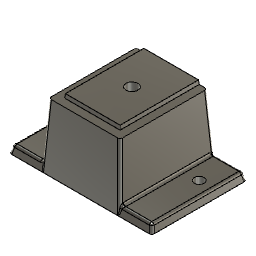
Mounting Base (Autodesk Fusion 360 design; units mm, degrees)
Autodesk Fusion 360 part; units mm, degrees
sketch "bottom" plane through (0, 0, 0) normal (0, 0, 1) x (1, 0, 0)
  line L0 (0, 0) -> (114.3, 0)
  line L1 (114.3, 0) -> (114.3, 76.2)
  line L2 (114.3, 76.2) -> (0, 76.2)
  line L3 (0, 76.2) -> (0, 0)
  line L4 (25.4, 76.2) -> (25.4, 0)
  line L5 (88.9, 0) -> (88.9, 76.2)
  line L6 (82.55, 6.35) -> (31.75, 6.35)
  line L7 (31.75, 69.85) -> (82.55, 69.85)
  line L8 (31.75, 69.85) -> (31.75, 6.35)
  line L9 (82.55, 6.35) -> (82.55, 69.85)
  circle A0 centre (12.7, 50.8) radius 3.9687
  circle A1 centre (101.6, 50.8) radius 3.9688
  dimension "d1" = 114.3
  dimension "d2" = 76.2
  dimension "d3" = 25.4
  dimension "d4" = 25.4
  dimension "d5" = 6.35
  dimension "d6" = 6.35
  dimension "d7" = 6.35
  dimension "d8" = 6.35
  dimension "d32" = 7.9375
  dimension "d33" = 7.9375
  dimension "d34" = 25.4
  dimension "d35" = 25.4
  dimension "d36" = 12.7
  dimension "d37" = 12.7
  constraint horizontal L0
  constraint vertical L1
  constraint horizontal L2
  constraint vertical L3
  constraint coincident L0.start L3.end
  constraint coincident L2 L4.start
  constraint coincident L0 L4.end
  constraint perpendicular L0 L4
  constraint coincident L0 L5.start
  constraint coincident L2 L5.end
  constraint perpendicular L2 L5
  constraint perpendicular L4 L6
  constraint perpendicular L5 L7
  constraint perpendicular L6 L8
  constraint perpendicular L7 L9
  measures "d1" distance of L0.start L0.end
  measures "d2" distance of L0.start L2.end
  measures "d3" distance of L3 L4
  measures "d4" distance of L1 L5
  measures "d5" distance of L2 L7
  measures "d6" distance of L0 L6
  measures "d7" distance of L4 L8
  measures "d8" distance of L5 L9
  measures "d32" diameter of A0
  measures "d33" diameter of A1
  measures "d34" distance of L2 A0.centre
  measures "d35" distance of L2 A1.centre
  measures "d36" distance of L3 A0.centre
  measures "d37" distance of L1 A1.centre
ref_plane "WorkPlane1" through (0, 0, 50.8) normal (0, 0, 1) x (1, 0, 0)
sketch "top" plane through (0, 0, 50.8) normal (0, 0, 1) x (1, 0, 0)
  line L0 (28.575, 73.025) -> (28.575, 3.175)
  line L1 (85.725, 3.175) -> (85.725, 73.025)
  line L2 (28.575, 73.025) -> (85.725, 73.025)
  line L3 (28.575, 3.175) -> (85.725, 3.175)
  line L4 (79.375, 73.025) -> (79.375, 9.525)
  line L5 (34.925, 73.025) -> (34.925, 9.525)
  line L6 (34.925, 9.525) -> (79.375, 9.525)
  circle A0 centre (57.15, 41.275) radius 4.7625
  dimension "d20" = 6.35
  dimension "d21" = 44.45
  dimension "d22" = 6.35
  dimension "d25" = 9.525
  dimension "d26" = 38.1
  dimension "d27" = 22.225
  constraint perpendicular L1 L2
  constraint perpendicular L1 L3
  constraint coincident L2 L4.start
  constraint perpendicular L3 L4
  constraint coincident L2 L5.start
  constraint perpendicular L3 L5
  constraint perpendicular L4 L6
  measures "d20" distance of L1 L4
  measures "d21" distance of L4 L5
  measures "d22" distance of L3 L6
  measures "d25" diameter of A0
  measures "d26" distance of L3 A0.centre
  measures "d27" distance of L5 A0.centre
ref_plane "WorkPlane2" through (0, 0, 44.45) normal (0, 0, 1) x (1, 0, 0)
sketch "top of hole" plane through (0, 0, 44.45) normal (0, 0, 1) x (1, 0, 0)
  line L0 (34.925, 66.675) -> (34.925, 9.525)
  line L1 (34.925, 9.525) -> (79.375, 9.525)
  line L2 (79.375, 9.525) -> (79.375, 66.675)
  line L3 (34.925, 66.675) -> (79.375, 66.675)
loft "Loft1" add profiles "top", "bottom" section 1 contours L0 L1 L2 L3 L4 L5 L6 | L2 L4 L5 L6 | A0 section 2 contours L0 L2 L4 L5 | L6 L7 L8 L9 makes body 1
extrude "Extrude1" add sketch "bottom" along normal blind 6.35 draft -14 separate body contours L0 L2 L3 L4 | L0 L2 L4 L5 | L0 L1 L2 L5 | L6 L7 L8 L9 | A0 | A1 makes body 2
loft "Loft2" cut profiles "bottom", "top of hole" section 1 contours L6 L7 L8 L9 section 2 bodies 1 2
extrude "Extrude2" add sketch "top" along normal blind 3.175 draft -5 separate body contours L2 L4 L5 L6 | A0 makes body 3
extrude "Extrude3" cut sketch "top" along normal up to surface (3.175 mm away) contours A0 bodies 3
extrude "Extrude4" cut sketch "top" against normal up to surface (6.35 mm away) contours A0 bodies 1
extrude "Extrude5" cut sketch "bottom" along normal up to surface (6.35 mm away) contours A0 bodies 2
extrude "Extrude6" cut sketch "bottom" along normal up to surface (6.35 mm away) contours A1 bodies 2
combine "Combine1" operation add target body 1 tool bodies 2 3
fillet "Fillet2" radius 2 1 edges at (25.7969, 38.1, 6.35) on bodies 1
fillet "Fillet3" radius 2 5 edges at (12.7506, 74.6168, 6.35) (25.2874, 74.4815, 6.8923) (1.5832, 38.1, 6.35) (25.2874, 1.7185, 6.8923) (12.7506, 1.5832, 6.35) on bodies 1
fillet "Fillet4" radius 2 1 edges at (26.9875, 1.5875, 25.4) on bodies 1
fillet "Fillet5" radius 2 5 edges at (0.6026, 0.6026, 2.4169) (1.9145, 1.9145, 5.926) (0.6026, 75.5974, 2.4169) (1.9145, 74.2855, 5.926) (26.9875, 74.6125, 25.4) on bodies 1
fillet "Fillet6" radius 2 1 edges at (87.3125, 1.5875, 25.4) on bodies 1
fillet "Fillet7" radius 2 1 edges at (87.3125, 74.6125, 25.4) on bodies 1
fillet "Fillet8" radius 2 3 edges at (100.5244, 74.6168, 6.35) (112.7168, 38.1, 6.35) (100.5244, 1.5832, 6.35) on bodies 1
fillet "Fillet9" radius 2 4 edges at (113.6974, 75.5974, 2.4169) (112.3855, 74.2855, 5.926) (113.6974, 0.6026, 2.4169) (112.3855, 1.9145, 5.926) on bodies 1
fillet "Fillet10" radius 2 7 edges at (87.7739, 0.3205, 1.2855) (88.4126, 1.6296, 5.6539) (88.5055, 2.7573, 6.3119) (88.5031, 38.1, 6.35) (88.5055, 73.4427, 6.3119) (88.4126, 74.5704, 5.6539) (87.7739, 75.8795, 1.2855) on bodies 1
